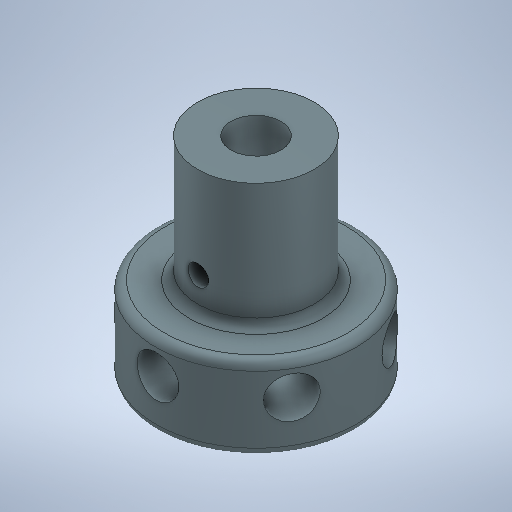
# Autodesk Inventor part: 22.4
Saved by Autodesk Inventor 2025.1 (Build 291241000, 241)
## iProperties
Created: 2024-09-13
Part Number: 22.4
Material: Lead
Document SubType Name: Modeling
Designer: ffogue
Density: 11.34 g/cm^3
Appearance: Lead
Author: ffogue
Autodesk Inventor part; units mm, degrees
ref_plane "YZ Plane" through (0, 0, 0) normal (1, 0, 0) x (0, 1, 0)
sketch "Sketch1" plane through (0, 0, 0) normal (0, 0, 1) x (1, 0, 0)
  circle A0 centre (0, 0) radius 12
  dimension "d0" = 24
  constraints: 1 centre point, 1 coincident
  measures "d0" diameter of A0
extrude "Extrusion1" add sketch "Sketch1" against normal blind 10
sketch "Sketch2" plane through (0, 0, 0) normal (0, 0, 1) x (1, 0, 0)
  circle A0 centre (0, 0) radius 7
  dimension "d3" = 14
  constraints: 1 centre point, 1 coincident
  measures "d3" diameter of A0
extrude "Extrusion2" add sketch "Sketch2" along normal blind 15
fillet "Fillet1" radius 1 3 edges at (-7, 0, 0) (-12, 0, 0) (-12, 0, -10)
ref_plane "Work Plane1" through (0, 12, 0) normal (0, 1, 0) x (-1, 0, 0)
sketch "Sketch4" plane through (0, 12, 0) normal (0, 1, 0) x (-1, 0, 0)
  line L0 (11, -10) -> (-11, -10) projected
  point P0 (0, 0)
  point P1 (0, -4)
  dimension "d15" = 6
  constraints: 1 vertical alignment
  measures "d15" distance from line of L0 point (0, -4)
hole "Hole2" at (0, 12, -4) direction (0, -1, 0) diameter 5 depth 8
pattern_circular "Circular Pattern1" count 6 over 360 about axis through (0, 0, -9) along (0, 0, -1) of "Hole2"
ref_plane "Work Plane2" through (0, 7, 0) normal (0, 1, 0) x (-1, 0, 0)
sketch "Sketch5" plane through (0, 7, 0) normal (0, 1, 0) x (-1, 0, 0)
  line L0 (7, 15) -> (-7, 15) projected
  line L1 (2.3094, -4.9574) -> (2.3094, -3.0426) projected
  arc A0 (2.3094, -3.0426) -> (-2.3094, -3.0426) centre (0, -4) ccw projected
  line L2 (-2.3094, -3.0426) -> (-2.3094, -4.9574) projected
  arc A1 (-2.3094, -4.9574) -> (2.3094, -4.9574) centre (0, -4) ccw projected
  point P0 (0, 0)
  point P1 (0, 4)
  point P2 (0, -6.5)
  point P3 (0, -1.5)
  point P4 (0, -3.5)
  point P5 (0, -8.5)
  point P6 (0, -2.5)
  point P7 (0, -7.5)
  dimension "d27" = 11
  constraints: 1 vertical alignment, 2 other
  measures "d27" distance from line of L0 point (0, 4)
hole "Hole3" at (0, 7, 4) direction (0, -1, 0) diameter 2.459 end through all thread size "M3x0.5" class "6H" standard "ISO Metric profile"
sketch "Sketch6" plane through (0, 0, 15) normal (0, 0, 1) x (1, 0, 0)
  circle A0 centre (0, 0) radius 7 projected
  constraints: 1 coincident
hole "Hole4" at (0, 0, 15) direction (0, 0, -1) diameter 6 depth 25
body "Solid1"
